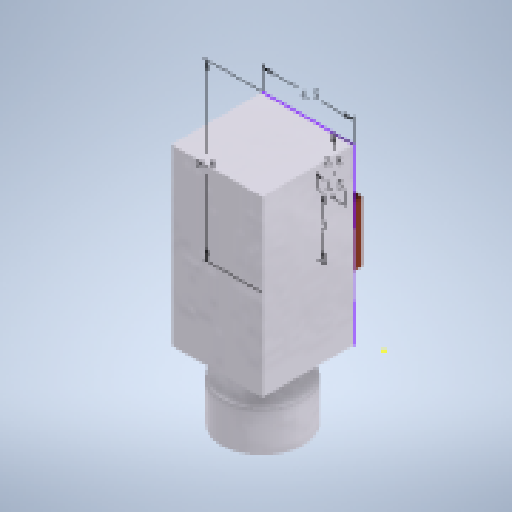
# Autodesk Inventor part: mortor
Saved by Autodesk Inventor 2025 (Build 290162000, 162)
## iProperties
Created: 2024-09-21
Part Number: mortor
Material: 常规
Document SubType Name: Modeling
Designer: shila
Density: 1 g/cm^3
Appearance: 银
Author: shila
Autodesk Inventor part; units mm, degrees
ref_plane "YZ Plane" through (0, 0, 0) normal (1, 0, 0) x (0, 1, 0)
ref_plane "XZ Plane" through (0, 0, 0) normal (0, 1, 0) x (-1, 0, 0)
ref_plane "XY Plane" through (0, 0, 0) normal (0, 0, 1) x (1, 0, 0)
sketch "草图1" plane through (0, 0, 0) normal (0, 0, 1) x (1, 0, 0)
  line L0 (-6.0016, 8.0804) -> (-1.5016, 8.0804)
  line L1 (-1.5016, 8.0804) -> (-1.5016, -0.5196)
  line L2 (-1.5016, -0.5196) -> (-6.0016, -0.5196)
  line L3 (-6.0016, -0.5196) -> (-6.0016, 8.0804)
  line L4 (-3.7516, 8.0804) -> (-3.7516, -0.5196)
  line L5 (-3.3516, 5.2804) -> (-1.8516, 5.2804)
  line L6 (-1.8516, 5.2804) -> (-1.8516, 2.2804)
  line L7 (-1.8516, 2.2804) -> (-3.3516, 2.2804)
  line L8 (-3.3516, 2.2804) -> (-3.3516, 5.2804)
  line L9 (-4.1516, 5.2804) -> (-5.6516, 5.2804)
  line L10 (-5.6516, 5.2804) -> (-5.6516, 2.2804)
  line L11 (-5.6516, 2.2804) -> (-4.1516, 2.2804)
  line L12 (-4.1516, 2.2804) -> (-4.1516, 5.2804)
  point P0 (0, 0)
  dimension "d0" = 4.5
  dimension "d1" = 8.6
  dimension "d5" = 1.5
  dimension "d6" = 3
  dimension "d7" = 2.8
  constraints: 26 end point, 4 parallel, 4 symmetric about line, 2 midpoint, 2 perpendicular, 1 horizontal
  measures "d0" distance of L0.start L0.end
  measures "d1" distance of L2.end L0.start
  measures "d5" distance of L5.start L5.end
  measures "d6" distance of L7.end L5.start
  measures "d7" vertical distance of L5.end L0.end
extrude "拉伸1" add sketch "草图1" along normal blind 4.5 contours L0 L4 L2 L3 | L0 L1 L2 L4 | L5 L6 L7 L8 | L12 L11 L10 L9
extrude "拉伸2" add sketch "草图1" against normal blind 0.8 contours L5 L6 L7 L8 | L12 L11 L10 L9
sketch "草图2" plane through (-6.0016, -0.5196, 0) normal (0, -1, 0) x (1, 0, 0)
  line L0 (0, 4.5) -> (4.5, 4.5) projected
  line L1 (2.25, 4.5) -> (2.25, 0)
  line L2 (4.5, 0) -> (0, 0) projected
  line L3 (4.5, 0) -> (4.5, 4.5) projected
  line L4 (4.5, 2.25) -> (0, 2.25)
  line L5 (0, 0) -> (0, 4.5) projected
  circle A0 centre (2.25, 2.25) radius 1.15
  point P0 (6.0016, 0)
  dimension "d10" = 2.3
  constraints: 5 midpoint, 4 end point, 1 centre point
  measures "d10" diameter of A0
extrude "拉伸3" add sketch "草图2" along normal blind 1 contours A0 L4 L1 | L1 L4 A0 | L4 L1 A0 | L4 A0 L1
sketch "草图3" plane through (-3.7516, -1.5196, 2.25) normal (0, -1, 0) x (1, 0, 0)
  circle A0 centre (0, 0) radius 0.5
  point P0 (3.7516, -2.25)
  dimension "d13" = 1
  constraints: 1 centre point
  measures "d13" diameter of A0
extrude "拉伸4" add sketch "草图3" along normal blind 2.3
sketch "草图4" plane through (-3.7516, -3.8196, 2.25) normal (0, -1, 0) x (1, 0, 0)
  circle A0 centre (0, 0) radius 2
  point P0 (3.7516, -2.25)
  dimension "d16" = 4
  constraints: 1 centre point
  measures "d16" diameter of A0
extrude "拉伸5" add sketch "草图4" against normal blind 2
